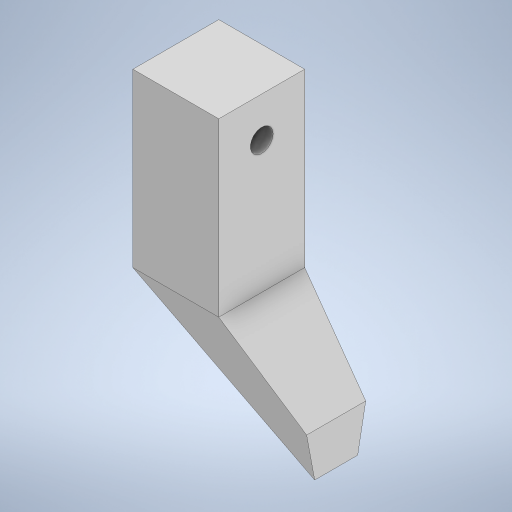
# Autodesk Inventor part: Gripper
Saved by Autodesk Inventor 2024 (Build 280153000, 153)
## iProperties
Created: 2025-01-21
Part Number: Gripper
Material: Generic
Document SubType Name: Modeling
Designer: Sven
Density: 1 g/cm^3
Appearance: Default
Author: Sven
Autodesk Inventor part; units mm, degrees
ref_plane "YZ Plane" through (0, 0, 0) normal (1, 0, 0) x (0, 1, 0)
ref_plane "XZ Plane" through (0, 0, 0) normal (0, 1, 0) x (-1, 0, 0)
ref_plane "XY Plane" through (0, 0, 0) normal (0, 0, 1) x (1, 0, 0)
sketch "Sketch1" plane through (0, 0, 0) normal (0, 0, 1) x (1, 0, 0)
  line L0 (-38.1, 76.2) -> (0, 76.2)
  line L1 (0, 76.2) -> (0, 0)
  line L2 (0, 0) -> (-38.1, 0)
  line L3 (-38.1, 0) -> (-38.1, 76.2)
  line L4 (-38.1, 0) -> (33.02, -50.8)
  line L5 (33.02, -50.8) -> (33.02, -31.75)
  line L6 (33.02, -31.75) -> (0, 0)
  dimension "d0" = 76.2
  dimension "d1" = 38.1
  dimension "d3" = 71.12
  dimension "d4" = 50.8
  dimension "d5" = 19.05
  dimension "d12" = 33.02
  constraints: 14 end point, 2 parallel, 1 coincident, 1 horizontal, 1 perpendicular, 1 vertical
  measures "d0" distance of L2.end L0.start
  measures "d1" distance of L0.start L0.end
  measures "d3" horizontal distance of L2.end L4.end
  measures "d4" vertical distance of L4.end point (0, 0)
  measures "d5" distance of L4.end L5.end
  measures "d12" distance from line of L5.end L1
extrude "Extrusion1" add sketch "Sketch1" along normal blind 38.1
sketch "Sketch3" plane through (-38.1, 0, 0) normal (-1, 0, 0) x (0, 0, 1)
  line L0 (0, 76.2) -> (38.1, 76.2) construction
  line L1 (19.05, 76.2) -> (19.05, -59.6946) construction
  line L2 (0, -31.75) -> (0, 0) projected
  line L3 (0, 0) -> (0, -50.8)
  line L4 (0, -50.8) -> (9.525, -50.8)
  line L5 (9.525, -50.8) -> (0, 0)
  line L6 (0, -50.8) -> (38.1, -50.8) projected
  line L7 (38.1, 0) -> (38.1, -50.8)
  line L8 (38.1, -50.8) -> (28.575, -50.8)
  line L9 (28.575, -50.8) -> (38.1, 0)
  point P0 (38.1, -31.75)
  point P1 (38.1, -50.8)
  point P2 (0, -31.75)
  dimension "d9" = 9.525
  constraints: 14 end point, 4 symmetric about line, 2 vertical, 1 collinear, 1 midpoint, 1 perpendicular
  measures "d9" distance from line of L1 L4.end
extrude "Extrusion2" cut sketch "Sketch3" against normal up to surface (71.12 mm away)
sketch "Sketch4" plane through (0, 76.2, 38.1) normal (1, 0, 0) x (0, 0, -1)
  circle A0 centre (19.05, -17.78) radius 5.05
  line L0 (38.1, 0) -> (0, 0) projected
  point P0 (38.1, -76.2)
  point P1 (19.05, 0)
  dimension "d13" = 10.1
  dimension "d14" = 17.78
  constraints: 1 centre point, 1 midpoint, 1 vertical alignment
  measures "d13" diameter of A0
  measures "d14" distance from line of L0 A0.centre
extrude "Extrusion3" cut sketch "Sketch4" against normal up to surface (38.1 mm away)
body "Solid1"
